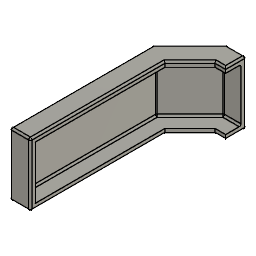
case left v12 (Autodesk Fusion 360 design; units mm, degrees)
Autodesk Fusion 360 part; units mm, degrees
sketch "Sketch1" plane through (0, 0, 0) normal (0, 0, 1) x (1, 0, 0)
  line L0 (0, 0) -> (0, 80) construction
  line L1 (0, 80) -> (20, 100) construction
  line L2 (20, 100) -> (30, 100) construction
  line L3 (9, 0) -> (9, 76.2721)
  line L4 (9, 76.2721) -> (23.7279, 91)
  line L5 (23.7279, 91) -> (30, 91)
  line L6 (-3, 0) -> (-3, 81.2426)
  line L7 (-3, 81.2426) -> (18.7574, 103)
  line L8 (18.7574, 103) -> (30, 103)
  line L9 (0, 0) -> (9, 0) construction
  line L10 (0, 0) -> (-3, 0) construction
  line L11 (30, 100) -> (30, 91)
  line L12 (30, 100) -> (30, 103)
  line L13 (0, -3) -> (9, -3)
  line L14 (0, -3) -> (-3, -3)
  line L15 (9, -3) -> (9, 0)
  line L16 (-3, -3) -> (-3, 0)
  dimension "d7" = 80
  dimension "d8" = 135
  dimension "d9" = 100
  dimension "d10" = 10
  dimension "d11" = 9
  dimension "d12" = -3
  dimension "d13" = 3
  constraint coincident L0.start L9.start
  constraint vertical L0
  constraint perpendicular L0 L2
  constraint perpendicular L3 L9
  constraint perpendicular L6 L10
  constraint perpendicular L5 L11
  constraint perpendicular L8 L12
  constraint perpendicular L9 L15
  constraint perpendicular L10 L16
  measures "d7" distance of L0.start L0.end
  measures "d8" angle of L0 L1
  measures "d9" vertical distance of L0.start L1.end
  measures "d10" distance of L1.end L2.end
extrude "Extrude1" add sketch "Sketch1" along normal blind 37.22
shell "Shell1" thickness 3 removed faces 6 at (30, 101, 12.4067) at (30, 97, 24.8133) at (25.8186, 91, 12.4067) at (13.9093, 81.1814, 24.8133) at (9, -2, 12.4067) at (9, 25.424, 12.4067)
fillet "Fillet2" radius 1 2 edges at (25, 100, 34.22) (25, 100, 3) 8 faces at (0, 53.3333, 23.8133) (6.6667, 86.6667, 13.4067) (1, -3, 12.4067) (1, 51.5049, 37.22) (22.5049, 103, 24.8133) (4.2525, 88.4951, 12.4067) (1, 51.5049, 0) (-3, 53.1618, 24.8133)
